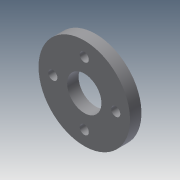
# Autodesk Inventor part: otoc. kruh, lozisko
Saved by Autodesk Inventor 2013 (Build 170138000, 138)
## iProperties
Created: 2013-05-11
Part Number: otoc. kruh, lozisko
Material: Generic
Document SubType Name: Modeling
Designer: idle-rug
Density: 1 g/cm^3
Author: idle-rug
Autodesk Inventor part; units mm, degrees
ref_plane "YZ Plane" through (0, 0, 0) normal (1, 0, 0) x (0, 1, 0)
ref_plane "XZ Plane" through (0, 0, 0) normal (0, 1, 0) x (-1, 0, 0)
ref_plane "XY Plane" through (0, 0, 0) normal (0, 0, 1) x (1, 0, 0)
sketch "Sketch1" plane through (0, 0, 0) normal (0, 1, 0) x (-1, 0, 0)
  circle A0 centre (0, 0) radius 20
  circle A1 centre (0, 0) radius 7.5
  line L0 (0, -7.5) -> (0, -20)
  circle A2 centre (0, -13.75) radius 2
  circle A3 centre (13.75, 0) radius 2
  circle A4 centre (-13.75, 0) radius 2
  circle A5 centre (0, 13.75) radius 2
  dimension "d3" = 15
  dimension "d8" = 4
  dimension "d9" = 4
  dimension "d10" = 4
  dimension "d11" = 4
  constraints: 4 centre point, 2 end point, 2 vertical alignment, 1 coincident, 1 midpoint, 1 point on line, 1 vertical, 4 other
  measures "d8" diameter of A2
  measures "d9" diameter of A3
  measures "d10" diameter of A4
  measures "d11" diameter of A5
extrude "Extrusion1" add sketch "Sketch1" along normal blind 5
body "Solid1"
